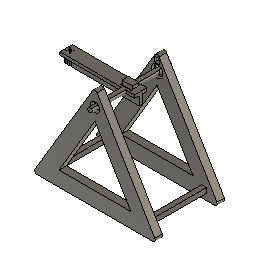
FLYArm-1D (Autodesk Fusion 360 design; units mm, degrees)
Autodesk Fusion 360 part; units mm, degrees
sketch "Szkic1" plane through (0, 0, 0) normal (0, 1, 0) x (1, 0, 0) in component "Base"
  line L0 (0, 0) -> (-250, 0)
  line L1 (-250, 0) -> (-250, -210)
  line L2 (-250, -210) -> (0, -210)
  line L3 (0, -210) -> (0, 0)
  line L4 (-250, 0) -> (-125, -210)
  line L5 (0, 0) -> (-125, -210)
  line L6 (-197.2304, -30) -> (-125, -151.3471)
  line L7 (-52.7696, -30) -> (-125, -151.3471)
  line L8 (-52.7696, -30) -> (-197.2304, -30)
  circle A0 centre (-125, -200.2245) radius 5
  circle A1 centre (-8.7949, -5) radius 5
  circle A2 centre (-241.2051, -5) radius 5
  circle A3 centre (-125, -175.7858) radius 12.025
  line L9 (-197.2304, -30) -> (-241.2051, -5)
  line L10 (-214.2178, -12.5) -> (-224.2178, -12.5)
  line L11 (-224.2178, -12.5) -> (-224.2178, -22.5)
  line L12 (-224.2178, -22.5) -> (-214.2178, -22.5)
  line L13 (-214.2178, -22.5) -> (-214.2178, -12.5)
  line L14 (-214.2178, -12.5) -> (-224.2178, -22.5) construction
  line L15 (-224.2178, -12.5) -> (-214.2178, -22.5) construction
  line L16 (-52.7696, -30) -> (-8.7949, -5)
  line L17 (-25.7822, -22.5) -> (-35.7822, -22.5)
  line L18 (-35.7822, -22.5) -> (-35.7822, -12.5)
  line L19 (-35.7822, -12.5) -> (-25.7822, -12.5)
  line L20 (-25.7822, -12.5) -> (-25.7822, -22.5)
  line L21 (-25.7822, -22.5) -> (-35.7822, -12.5) construction
  line L22 (-35.7822, -22.5) -> (-25.7822, -12.5) construction
  circle A4 centre (-125, -175.7858) radius 9.525
  line L23 (-125, -175.7858) -> (-112.975, -175.7858)
  line L24 (-125, -175.7858) -> (-137.025, -175.7858)
  line L25 (-125, -200.2245) -> (-125, -195.2245)
  line L26 (-125, -195.2245) -> (-125, -194.2245)
  line L27 (-120, -189.2245) -> (-130, -189.2245)
  line L28 (-130, -189.2245) -> (-130, -199.2245)
  line L29 (-130, -199.2245) -> (-120, -199.2245)
  line L30 (-120, -199.2245) -> (-120, -189.2245)
  line L31 (-120, -189.2245) -> (-130, -199.2245) construction
  line L32 (-130, -189.2245) -> (-120, -199.2245) construction
  point P0 (-219.2178, -17.5)
  point P1 (-30.7822, -17.5)
  point P2 (-125, -194.2245)
  point P3 (-125, -194.2245)
  dimension "d1" = 250
  dimension "d2" = 210
  dimension "d7" = 5
  dimension "d8" = 5
  dimension "d9" = 5
  dimension "d18" = 24.05
  dimension "d19" = 10
  dimension "d20" = 10
  dimension "d21" = 10
  dimension "d22" = 10
  dimension "d28" = 19.05
  dimension "d115" = 1
  dimension "d121" = 10
  dimension "d122" = 10
  constraint horizontal L0
  constraint vertical L1
  constraint horizontal L2
  constraint vertical L3
  constraint coincident L0.start L3.end
  constraint midpoint L2 L4.end
  constraint tangent L4 A0
  constraint tangent L5 A0
  constraint tangent L0 A1
  constraint tangent L5 A1
  constraint tangent L4 A2
  constraint tangent L0 A2
  constraint coincident A2.centre L9.end
  constraint horizontal L10
  constraint perpendicular L10 L11
  constraint parallel L10 L12
  constraint parallel L11 L13
  constraint coincident L14 P0
  constraint coincident L15 P0
  constraint midpoint L9 P0
  constraint coincident A1.centre L16.end
  constraint horizontal L17
  constraint perpendicular L17 L18
  constraint parallel L17 L19
  constraint parallel L18 L20
  constraint coincident L21 P1
  constraint coincident L22 P1
  constraint midpoint L16 P1
  constraint concentric A3 A4
  constraint coincident A3.centre A4.centre
  constraint coincident A3 L23.end
  constraint coincident A3 L24.end
  constraint coincident A0.centre L25.start
  constraint coincident A0 L25.end
  constraint vertical L25
  constraint parallel L25 L26
  constraint coincident P3 P2
  constraint horizontal L27
  constraint perpendicular L27 L28
  constraint parallel L27 L29
  constraint parallel L28 L30
  constraint coincident L31 P3
  constraint coincident L32 P3
  measures "d1" distance of L0.start L0.end
  measures "d2" distance of L0.start L2.end
  measures "d7" radius of A0
  measures "d8" radius of A1
  measures "d9" radius of A2
  measures "d18" diameter of A3
  measures "d19" distance of L11.end L12.end
  measures "d20" distance of L10.end L11.end
  measures "d21" distance of L18.end L19.end
  measures "d22" distance of L17.end L18.end
  measures "d28" diameter of A4
  measures "d115" distance of L25.end P3
  measures "d121" distance of L28.end L29.end
  measures "d122" distance of L27.end L28.end
extrude "Wyciągnięcie proste4" add sketch "Szkic1" against normal blind 10 contours L0 L8 A1 A2 L9 L10 L11 L13 L16 L18 L19 L20 | A1 | L4 L5 L6 L7 A0 A1 A2 L9 L11 L12 L13 L16 L17 L18 L20 L27 L28 L29 L30 | A2 | A0 L29 | L16 L17 L18 L20 | L16 L18 L19 L20 | A0 L27 L28 L29 L30 | A0 L25 L29 | A0 L25 L29 | L9 L10 L11 L13 | L9 L11 L12 L13 | A3 A4 L23 L24 | A3 A4 L23 L24 | A4 L23 L24 | A4 L23 L24 makes body 1 in component "Base"
extrude "Wyciągnięcie proste5" cut sketch "Szkic1" against normal blind 7 contours L16 L17 L18 L20 | L16 L18 L19 L20 | A0 L27 L28 L29 L30 | A0 L25 L29 | A0 L25 L29 | L9 L10 L11 L13 | L9 L11 L12 L13 | A3 A4 L23 L24 | A3 A4 L23 L24 bodies 1 in component "Base"
extrude "Wyciągnięcie proste6" cut sketch "Szkic1" against normal blind 10 contours A4 L23 L24 | A4 L23 L24 bodies 1 in component "Base"
sketch "Szkic1 (2)" plane through (0, 0, 0) normal (0, 0, 1) x (1, 0, 0) in component "Connector"
  line L0 (0, 0) -> (9.9, 0)
  line L1 (9.9, 0) -> (9.9, 124)
  line L2 (9.9, 124) -> (0, 124)
  line L3 (0, 124) -> (0, 0)
  dimension "d41" = 9.9
  dimension "d42" = 124
  constraint horizontal L0
  constraint vertical L1
  constraint horizontal L2
  constraint vertical L3
  constraint coincident L0.start L3.end
  measures "d41" distance of L0.start L0.end
  measures "d42" distance of L0.start L2.end
extrude "Wyciągnięcie proste1" add sketch "Szkic1 (2)" along normal blind 9.9 separate body makes body 2 in component "Connector"
other "Zależność geometryczna4"
other "Zależność geometryczna5"
other "Zależność geometryczna6"
other "Zależność geometryczna7"
other "Zależność geometryczna8"
other "Zależność geometryczna9"
sketch "Szkic1 (3)" plane through (0, 0, 0) normal (0, 1, 0) x (1, 0, 0) in component "Base2"
  line L0 (0, 0) -> (-250, 0)
  line L1 (-250, 0) -> (-250, -210)
  line L2 (-250, -210) -> (0, -210)
  line L3 (0, -210) -> (0, 0)
  line L4 (0, 0) -> (-125, -210)
  line L5 (-125, -210) -> (-250, 0)
  line L6 (-52.7696, -30) -> (-125, -151.3471)
  line L7 (-125, -151.3471) -> (-197.2304, -30)
  line L8 (-52.7696, -30) -> (-197.2304, -30)
  circle A0 centre (-125, -200.2245) radius 5
  circle A1 centre (-241.2051, -5) radius 5
  circle A2 centre (-8.7949, -5) radius 5
  line L9 (-241.2051, -5) -> (-197.2304, -30)
  line L10 (-8.7949, -5) -> (-52.7696, -30)
  circle A3 centre (-125, -175.7858) radius 12.025
  circle A4 centre (-125, -175.7858) radius 9.525
  line L11 (-35.7822, -12.5) -> (-25.7822, -12.5)
  line L12 (-25.7822, -12.5) -> (-25.7822, -22.5)
  line L13 (-25.7822, -22.5) -> (-35.7822, -22.5)
  line L14 (-35.7822, -22.5) -> (-35.7822, -12.5)
  line L15 (-35.7822, -12.5) -> (-25.7822, -22.5) construction
  line L16 (-25.7822, -12.5) -> (-35.7822, -22.5) construction
  line L17 (-224.2178, -22.5) -> (-214.2178, -22.5)
  line L18 (-214.2178, -22.5) -> (-214.2178, -12.5)
  line L19 (-214.2178, -12.5) -> (-224.2178, -12.5)
  line L20 (-224.2178, -12.5) -> (-224.2178, -22.5)
  line L21 (-224.2178, -22.5) -> (-214.2178, -12.5) construction
  line L22 (-214.2178, -22.5) -> (-224.2178, -12.5) construction
  line L23 (-125, -200.2245) -> (-125, -195.2245)
  line L24 (-125, -195.2245) -> (-125, -194.2245)
  line L25 (-130, -189.2245) -> (-120, -189.2245)
  line L26 (-120, -189.2245) -> (-120, -199.2245)
  line L27 (-120, -199.2245) -> (-130, -199.2245)
  line L28 (-130, -199.2245) -> (-130, -189.2245)
  line L29 (-130, -189.2245) -> (-120, -199.2245) construction
  line L30 (-120, -189.2245) -> (-130, -199.2245) construction
  point P0 (-30.7822, -17.5)
  point P1 (-219.2178, -17.5)
  point P2 (-125, -194.2245)
  dimension "d54" = 250
  dimension "d55" = 210
  dimension "d57" = 5
  dimension "d58" = 5
  dimension "d59" = 5
  dimension "d60" = 24.05
  dimension "d61" = 19.05
  dimension "d65" = 10
  dimension "d66" = 10
  dimension "d67" = 10
  dimension "d68" = 10
  dimension "d118" = 1
  dimension "d119" = 10
  dimension "d120" = 10
  constraint horizontal L0
  constraint vertical L1
  constraint horizontal L2
  constraint vertical L3
  constraint coincident L0.start L3.end
  constraint midpoint L2 L4.end
  constraint tangent L4 A0
  constraint tangent L5 A0
  constraint tangent L5 A1
  constraint tangent L0 A1
  constraint tangent L0 A2
  constraint tangent L4 A2
  constraint coincident A1.centre L9.start
  constraint coincident A2.centre L10.start
  constraint concentric A3 A4
  constraint horizontal L11
  constraint perpendicular L11 L12
  constraint parallel L11 L13
  constraint parallel L12 L14
  constraint coincident L15 P0
  constraint coincident L16 P0
  constraint midpoint L10 P0
  constraint horizontal L17
  constraint perpendicular L17 L18
  constraint parallel L17 L19
  constraint parallel L18 L20
  constraint coincident L21 P1
  constraint coincident L22 P1
  constraint midpoint L9 P1
  constraint coincident A0.centre L23.start
  constraint coincident A0 L23.end
  constraint vertical L23
  constraint parallel L23 L24
  constraint horizontal L25
  constraint perpendicular L25 L26
  constraint parallel L25 L27
  constraint parallel L26 L28
  constraint coincident L29 P2
  constraint coincident L30 P2
  constraint coincident P2 L24.end
  measures "d54" distance of L0.start L0.end
  measures "d55" distance of L0.start L2.end
  measures "d57" radius of A0
  measures "d58" radius of A1
  measures "d59" radius of A2
  measures "d60" diameter of A3
  measures "d61" diameter of A4
  measures "d65" distance of L12.end L13.end
  measures "d66" distance of L11.end L12.end
  measures "d67" distance of L18.end L19.end
  measures "d68" distance of L17.end L18.end
  measures "d118" distance of L23.end P2
  measures "d119" distance of L26.end L27.end
  measures "d120" distance of L25.end L26.end
  measures "d221" distance of L0.start
extrude "Wyciągnięcie proste1'" add sketch "Szkic1 (3)" along normal blind 10 separate body contours L0 L8 A1 A2 L9 L10 L11 L12 L14 L18 L19 L20 | A2 | L4 L5 L6 L7 A0 A1 A2 L9 L10 L12 L13 L14 L17 L18 L20 L25 L26 L27 L28 | A1 | A0 L27 | L10 L12 L13 L14 | L10 L11 L12 L14 | A0 L25 L26 L27 L28 | A0 L23 L27 | A0 L23 L27 | L9 L18 L19 L20 | L9 L17 L18 L20 | A3 | A4 makes body 3 in component "Base2"
extrude "Wyciągnięcie proste2" cut sketch "Szkic1 (3)" along normal blind 7 contours L10 L12 L13 L14 | L10 L11 L12 L14 | A0 L25 L26 L27 L28 | A0 L23 L27 | A0 L23 L27 | L9 L18 L19 L20 | L9 L17 L18 L20 | A3 bodies 3 in component "Base2"
extrude "Wyciągnięcie proste3" cut sketch "Szkic1 (3)" along normal blind 10 contours A4 bodies 3 in component "Base2"
other "Zależność geometryczna10"
other "Zależność geometryczna11"
other "Zależność geometryczna12"
ref_plane "Płaszczyzna konstrukcyjna1" through (-125, 0, 175.7858) normal (1, 0, 0) x (0, 1, 0) in component "Bar"
sketch "Szkic1 (4)" plane through (-125, 0, 175.7858) normal (1, 0, 0) x (0, 1, 0) in component "Bar"
  line L0 (0, 0) -> (95, 0)
  line L1 (47.5, 0) -> (60, 0)
  line L2 (47.5, 0) -> (35, 0)
  line L3 (60, 0) -> (60, -6)
  line L4 (35, 0) -> (35, -6)
  line L5 (47.5, 0) -> (47.5, -24)
  line L6 (47.5, -24) -> (50.5, -24)
  line L7 (47.5, -24) -> (44.5, -24)
  line L8 (50.5, -24) -> (50.5, -6)
  line L9 (44.5, -24) -> (44.5, -6)
  line L10 (35, -6) -> (44.5, -6)
  line L11 (60, -6) -> (50.5, -6)
  line L12 (95, 0) -> (95, -175.786)
  line L13 (0, 0) -> (0, -175.786)
  line L14 (0, -175.786) -> (95, -175.786)
  line L15 (47.5, -175.786) -> (47.5, -165.786)
  line L16 (47.5, -165.786) -> (47.5, -120.786)
  line L17 (47.5, -120.786) -> (47.5, 0)
  dimension "d82" = 12.5
  dimension "d83" = 12.5
  dimension "d85" = 6
  dimension "d86" = 6
  dimension "d91" = 24
  dimension "d92" = 3
  dimension "d93" = 3
  dimension "d94" = 18
  dimension "d95" = 18
  dimension "d99" = 175.786
  dimension "d100" = 175.786
  dimension "d102" = 10
  dimension "d103" = 45
  dimension "d104" = 120.786
  constraint coincident L0.start L13.start
  constraint horizontal L0
  constraint midpoint L0 L1.start
  constraint parallel L0 L1
  constraint parallel L0 L2
  constraint perpendicular L0 L3
  constraint perpendicular L2 L4
  constraint perpendicular L1 L5
  constraint perpendicular L5 L6
  constraint perpendicular L5 L7
  constraint perpendicular L6 L8
  constraint perpendicular L7 L9
  constraint perpendicular L0 L12
  constraint perpendicular L0 L13
  constraint midpoint L14 L15.start
  constraint perpendicular L14 L15
  constraint parallel L15 L16
  constraint perpendicular L2 L17
  measures "d82" distance of L1.start L1.end
  measures "d83" distance of L1.start L2.end
  measures "d85" distance of L1.end L3.end
  measures "d86" distance of L2.end L4.end
  measures "d91" distance of L1.start L5.end
  measures "d92" distance of L5.end L6.end
  measures "d93" distance of L5.end L7.end
  measures "d94" distance of L6.end L8.end
  measures "d95" distance of L7.end L9.end
  measures "d99" distance of L0.end L12.end
  measures "d100" distance of L0.start L13.end
  measures "d102" distance of L15.start L15.end
  measures "d103" distance of L15.end L16.end
  measures "d104" distance of L16.end L1.start
extrude "Wyciągnięcie proste1''" add sketch "Szkic1 (4)" against normal blind 128 separate body contours L0 L2 L4 L5 L7 L9 L10 L17 | L0 L1 L3 L5 L6 L8 L11 L17 makes body 4 in component "Bar"
sketch "Szkic2" plane through (0, 0, 175.7858) normal (0, 0, 1) x (-1, 0, 0) in component "Bar"
  line L0 (125, -60) -> (253, -60)
  line L1 (253, -60) -> (253, -35)
  line L2 (253, -35) -> (125, -35)
  line L3 (125, -47.5) -> (245, -47.5)
  line L4 (249.2425, -51.7425) -> (240.7575, -51.7425)
  line L5 (240.7575, -51.7425) -> (240.7575, -43.2575)
  line L6 (240.7575, -43.2575) -> (249.2425, -43.2575)
  line L7 (249.2425, -43.2575) -> (249.2425, -51.7425)
  line L8 (249.2425, -51.7425) -> (240.7575, -43.2575) construction
  line L9 (240.7575, -51.7425) -> (249.2425, -43.2575) construction
  circle A0 centre (240.7575, -43.2575) radius 1
  circle A1 centre (249.2425, -43.2575) radius 1
  circle A2 centre (240.7575, -51.7425) radius 1
  circle A3 centre (249.2425, -51.7425) radius 1
  circle A4 centre (245, -47.5) radius 2.5
  point P0 (245, -47.5)
  dimension "d152" = 120
  dimension "d153" = 8.485
  dimension "d154" = 8.485
  dimension "d155" = 2
  dimension "d156" = 2
  dimension "d157" = 2
  dimension "d158" = 2
  dimension "d191" = 5
  constraint horizontal L4
  constraint perpendicular L4 L5
  constraint parallel L4 L6
  constraint parallel L5 L7
  constraint coincident L8 P0
  constraint coincident L9 P0
  constraint coincident P0 L3.end
  constraint coincident L5.end L6.start
  constraint coincident L6.end L7.start
  constraint coincident L4.end L5.start
  constraint coincident L4.start L7.end
  measures "d152" distance of L3.start P0
  measures "d153" distance of L5.end L6.end
  measures "d154" distance of L4.end L5.end
  measures "d155" diameter of A0
  measures "d156" diameter of A1
  measures "d157" diameter of A2
  measures "d158" diameter of A3
  measures "d191" diameter of A4
other "Zależność geometryczna16"
other "Zależność geometryczna17"
other "Zależność geometryczna18"
extrude "Wyciągnięcie proste3'" add 1 faces at (-125, 47.5, 163.7858) along direction (1, 0, 0) blind 12.025 on bodies 4 bodies 4 in component "Bar"
ref_plane "Płaszczyzna konstrukcyjna2" through (-182.9875, 47.5, 172.7858) normal (0, 1, 0) x (0, 0, -1) in component "Bar"
sketch "Szkic5" plane through (0, 47.5, 0) normal (0, 1, 0) x (1, 0, 0) in component "Bar"
extrude "Wyciągnięcie proste8" cut sketch "Szkic2" against normal blind 36 contours L4 L5 A2 | L4 L5 A2 | L4 L7 A3 | L4 L7 A3 | L6 L7 A1 | L6 L7 A1 | L5 L6 A0 | L5 L6 A0 bodies 4 in component "Bar"
sketch "Szkic6" plane through (0, 50.5, 0) normal (0, 1, 0) x (-1, 0, 0) in component "Bar"
  line L0 (112.975, 151.7858) -> (253, 151.7858)
  line L1 (253, 151.7858) -> (253, 169.7858)
  line L2 (253, 169.7858) -> (112.975, 169.7858)
  line L3 (112.975, 169.7858) -> (112.975, 151.7858)
  line L4 (112.975, 169.7858) -> (125, 169.7858)
  line L5 (125, 169.7858) -> (125, 176.7858)
  line L6 (125, 169.7858) -> (125, 159.7858)
  circle A0 centre (125, 172.3108) radius 4.475
  line L7 (125, 176.7858) -> (125, 175.7858)
  line L8 (125, 175.7858) -> (122.1804, 175.7858)
  line L9 (125, 175.7858) -> (127.8196, 175.7858)
  line L10 (125, 176.7858) -> (125, 172.3108)
  circle A1 centre (125, 172.3108) radius 5.475
  line L11 (122.1804, 175.7858) -> (120.7692, 175.7858)
  line L12 (127.8196, 175.7858) -> (129.2308, 175.7858)
  dimension "d161" = 12.025
  dimension "d162" = 7
  dimension "d163" = 10
  dimension "d164" = 8.95
  dimension "d169" = 1
  dimension "d198" = 4.475
  dimension "d199" = 10.95
  constraint coincident L2.end L3.start
  constraint coincident L2 L4.end
  constraint perpendicular L2 L5
  constraint perpendicular L4 L6
  constraint coincident L5.end A0
  constraint parallel L5 L7
  constraint coincident A0 L8.end
  constraint perpendicular L7 L8
  constraint coincident A0 L9.end
  constraint perpendicular L7 L9
  constraint parallel L5 L10
  constraint concentric A0 A1
  constraint coincident A1 L11.end
  constraint parallel L8 L11
  constraint coincident A1 L12.end
  constraint parallel L9 L12
  measures "d161" distance of L2.end L4.end
  measures "d162" distance of L4.end L5.end
  measures "d163" distance of L4.end L6.end
  measures "d164" diameter of A0
  measures "d169" distance of L5.end L7.end
  measures "d198" distance of L5.end A0.centre
  measures "d199" diameter of A1
sketch "Szkic7" plane through (0, 44.5, 0) normal (0, -1, 0) x (1, 0, 0) in component "Bar"
  line L0 (-112.975, 169.7858) -> (-253, 169.7858)
  line L1 (-253, 169.7858) -> (-253, 151.7858)
  line L2 (-253, 151.7858) -> (-112.975, 151.7858)
  line L3 (-112.975, 151.7858) -> (-112.975, 169.7858)
  line L4 (-112.975, 169.7858) -> (-125, 169.7858)
  line L5 (-125, 169.7858) -> (-125, 176.7858)
  line L6 (-125, 169.7858) -> (-125, 159.7858)
  circle A0 centre (-125, 172.3108) radius 4.475
  line L7 (-125, 176.7858) -> (-125, 175.7858)
  line L8 (-125, 175.7858) -> (-122.1804, 175.7858)
  line L9 (-125, 175.7858) -> (-127.8196, 175.7858)
  line L10 (-125, 176.7858) -> (-125, 172.3108)
  circle A1 centre (-125, 172.3108) radius 5.475
  line L11 (-127.8196, 175.7858) -> (-129.2308, 175.7858)
  line L12 (-122.1804, 175.7858) -> (-120.7692, 175.7858)
  dimension "d165" = 12.025
  dimension "d166" = 7
  dimension "d167" = 10
  dimension "d168" = 8.95
  dimension "d170" = 1
  dimension "d202" = 4.475
  dimension "d203" = 10.95
  constraint coincident L0.start L3.end
  constraint perpendicular L3 L4
  constraint perpendicular L4 L5
  constraint perpendicular L4 L6
  constraint coincident L5.end A0
  constraint parallel L5 L7
  constraint coincident A0 L8.end
  constraint perpendicular L5 L8
  constraint coincident A0 L9.end
  constraint perpendicular L7 L9
  constraint perpendicular L8 L10
  constraint coincident A0.centre L10.end
  constraint coincident A1 L11.end
  constraint parallel L9 L11
  constraint coincident A1 L12.end
  constraint parallel L8 L12
  measures "d165" distance of L0.start L4.end
  measures "d166" distance of L4.end L5.end
  measures "d167" distance of L4.end L6.end
  measures "d168" diameter of A0
  measures "d170" distance of L5.end L7.end
  measures "d202" distance of L5.end A0.centre
  measures "d203" diameter of A1
extrude "Wyciągnięcie proste9" add sketch "Szkic7" along normal blind 77 contours L0 L4 L6 A0 | L0 L4 L5 A0 L8 L10 | L0 L6 A0 | L0 L5 A0 L9 L10 bodies 4 in component "Bar"
extrude "Wyciągnięcie proste10" add sketch "Szkic6" along normal blind 77 contours L2 L4 L5 A0 L8 L10 | L2 L4 L6 A0 | L2 L6 A0 | L2 L5 A0 L9 L10 bodies 4 in component "Bar"
sketch "Szkic11" plane through (0, 127.5, 0) normal (0, 1, 0) x (-1, 0, 0) in component "Bar"
  arc A0 (122.1804, 175.7858) -> (127.8196, 175.7858) centre (125, 172.3108) ccw
  line L0 (127.8196, 175.7858) -> (122.1804, 175.7858)
  circle A1 centre (125, 172.3108) radius 12.025
  line L1 (125, 172.3108) -> (125, 160.2858)
  line L2 (125, 172.3108) -> (125, 151)
  line L3 (125, 175.7858) -> (125, 169.7858)
  line L4 (125, 169.7858) -> (110.6889, 169.7858)
  line L5 (110.6889, 169.7858) -> (110.6889, 143)
  line L6 (125, 151) -> (105, 151)
  dimension "d181" = 24.05
  dimension "d182" = 6
  constraint concentric A0 A1
  constraint coincident A0.centre A1.centre
  constraint coincident A1 L1.end
  constraint vertical L1
  constraint parallel L1 L2
  constraint midpoint L0 L3.start
  constraint perpendicular L0 L3
  constraint perpendicular L1 L4
  constraint perpendicular L4 L5
  constraint perpendicular L2 L6
  measures "d181" diameter of A1
  measures "d182" distance of L3.start L3.end
extrude "Wyciągnięcie proste7" add 1 faces at (-149.0768, -10, 10) along direction (0, -1, 0) blind 5 on bodies 1 bodies 1 in component "Base"
extrude "Wyciągnięcie proste4'" add 1 faces at (-149.0768, 10, 10) along direction (0, 1, 0) blind 5 on bodies 3 bodies 3 in component "Base2"
other "Zależność geometryczna22"
extrude "Wyciągnięcie proste13" cut sketch "Szkic2" against normal blind 2 contours A4 bodies 4 in component "Bar"
sketch "Szkic12" plane through (0, 0, 175.7858) normal (0, 0, 1) x (-1, 0, 0) in component "Bar"
  circle A0 centre (245, -47.5) radius 2.5
  circle A1 centre (249.2425, -43.2575) radius 1
  circle A2 centre (240.7575, -43.2575) radius 1
  circle A3 centre (249.2425, -51.7425) radius 1
  circle A4 centre (240.7575, -51.7425) radius 1
  line L0 (127.8196, -60) -> (253, -60)
  line L1 (253, -60) -> (253, -35)
  line L2 (253, -35) -> (127.8196, -35)
  line L3 (127.8196, -35) -> (127.8196, 32.5)
  line L4 (127.8196, 32.5) -> (122.1804, 32.5)
  line L5 (122.1804, 32.5) -> (122.1804, -35)
  line L6 (122.1804, -35) -> (112.975, -35)
  line L7 (112.975, -35) -> (112.975, -60)
  line L8 (112.975, -60) -> (122.1804, -60)
  line L9 (122.1804, -60) -> (122.1804, -127.5)
  line L10 (122.1804, -127.5) -> (127.8196, -127.5)
  line L11 (127.8196, -127.5) -> (127.8196, -60)
  line L12 (122.1804, -35) -> (127.8196, -35)
  line L13 (122.1804, -35) -> (122.1804, -60)
  line L14 (125, -35) -> (125, -52.3294)
  line L15 (122.1804, -47.5) -> (129.8919, -47.5)
  line L16 (135.5, -39.5) -> (114.5, -39.5)
  line L17 (114.5, -39.5) -> (114.5, -55.5)
  line L18 (114.5, -55.5) -> (135.5, -55.5)
  line L19 (135.5, -55.5) -> (135.5, -39.5)
  line L20 (135.5, -39.5) -> (114.5, -55.5) construction
  line L21 (114.5, -39.5) -> (135.5, -55.5) construction
  point P0 (125, -47.5)
  dimension "d194" = 21
  dimension "d195" = 16
  constraint coincident L5.end L6.start
  constraint coincident L2.end L3.start
  constraint coincident L8.end L9.start
  constraint midpoint L12 L14.start
  constraint perpendicular L12 L14
  constraint midpoint L13 L15.start
  constraint perpendicular L13 L15
  constraint horizontal L16
  constraint perpendicular L16 L17
  constraint parallel L16 L18
  constraint parallel L17 L19
  constraint coincident L20 P0
  constraint coincident L21 P0
  constraint coincident L14 P0
  constraint coincident L15 P0
  measures "d194" distance of L17.end L18.end
  measures "d195" distance of L16.end L17.end
extrude "Wyciągnięcie proste14" add 1 faces at (-112.975, 46.5, 173.7858) along direction (1, 0, 0) blind 10 on bodies 4 bodies 4 in component "Bar"
extrude "Wyciągnięcie proste15" add sketch "Szkic6" along normal blind 52 contours L2 L4 A0 A1 L11 | L2 L4 L6 A0 A1 | L2 L6 A0 A1 | L2 A0 A1 L12 bodies 4 in component "Bar"
extrude "Wyciągnięcie proste16" add sketch "Szkic7" along normal blind 52 contours L0 L4 L6 A0 A1 | L0 L4 A0 A1 L12 | L0 L6 A0 A1 | L0 A0 A1 L11 bodies 4 in component "Bar"
other "Zależność geometryczna23"
sketch "Szkic13" plane through (0, 0, 169.7858) normal (0, 0, -1) x (1, 0, 0) in component "Bar"
  line L0 (-129.858, -60) -> (-129.858, -50.5)
  line L1 (-129.858, -50.5) -> (-253, -50.5)
  line L2 (-253, -50.5) -> (-253, -60)
  line L3 (-253, -60) -> (-129.858, -60)
  circle A0 centre (-249.2425, -51.7425) radius 1
  circle A1 centre (-240.7575, -51.7425) radius 1
  circle A2 centre (-240.7575, -51.7425) radius 2.5
  circle A3 centre (-249.2425, -51.7425) radius 2.5
  line L4 (-249.2425, -51.7425) -> (-240.7572, -43.2572)
  line L5 (-249.2425, -51.7425) -> (-237.2425, -51.7425) construction
  circle A4 centre (-240.7572, -43.2572) radius 2.5
  line L6 (-240.7575, -51.7425) -> (-249.2428, -43.2572)
  line L7 (-240.7575, -51.7425) -> (-252.7575, -51.7425) construction
  circle A5 centre (-249.2428, -43.2572) radius 2.5
  dimension "d207" = 5
  dimension "d208" = 5
  dimension "d209" = 45
  dimension "d210" = 12
  dimension "d211" = 5
  dimension "d212" = 45
  dimension "d213" = 12
  dimension "d214" = 5
  constraint concentric A1 A2
  constraint concentric A0 A3
  constraint horizontal L5
  constraint coincident A0.centre A3.centre
  constraint coincident L4.end A4.centre
  constraint horizontal L7
  constraint coincident A1.centre A2.centre
  constraint coincident L6.end A5.centre
  measures "d207" diameter of A2
  measures "d208" diameter of A3
  measures "d209" angle of L4 L5
  measures "d210" distance of A0.centre L4.end
  measures "d211" diameter of A4
  measures "d212" angle of L6 L7
  measures "d213" distance of A1.centre L6.end
  measures "d214" diameter of A5
extrude "Wyciągnięcie proste17" cut sketch "Szkic13" along normal blind 30 contours L1 A2 | L1 A2 L6 | L1 A2 L6 | L1 A3 L4 | L1 A3 | L1 A3 L4 | A4 | A5 bodies 4 in component "Bar"
extrude "Wyciągnięcie proste18" cut sketch "Szkic13" against normal blind 1.7 contours L1 A2 | L1 A2 L6 | L1 A2 L6 | L1 A3 L4 | L1 A3 | L1 A3 L4 | A4 | A5 bodies 4 in component "Bar"
extrude "Wyciągnięcie proste19" cut sketch "Szkic12" against normal blind 2 contours L13 L16 L17 L18 | L13 L14 L15 L16 L18 L19 | L13 L14 L15 L16 bodies 4 in component "Bar"
sketch "Szkic14" plane through (0, 0, 173.7858) normal (0, 0, 1) x (-1, 0, 0) in component "Bar"
  line L0 (135.5, -55.5) -> (135.5, -39.5)
  line L1 (135.5, -39.5) -> (114.5, -39.5)
  line L2 (114.5, -39.5) -> (114.5, -55.5)
  line L3 (114.5, -55.5) -> (135.5, -55.5)
  line L4 (114.5, -39.5) -> (135.5, -39.5)
  line L5 (135.5, -39.5) -> (135.5, -55.5)
  line L6 (135.5, -55.5) -> (114.5, -55.5)
  line L7 (114.5, -55.5) -> (114.5, -39.5)
  line L8 (125, -39.5) -> (125, -55.5)
  line L9 (125, -55.5) -> (125, -49)
  line L10 (135.35, -55.5) -> (114.65, -55.5)
  line L11 (114.65, -55.5) -> (114.65, -42.5)
  line L12 (114.65, -42.5) -> (135.35, -42.5)
  line L13 (135.35, -42.5) -> (135.35, -55.5)
  line L14 (135.35, -55.5) -> (114.65, -42.5) construction
  line L15 (114.65, -55.5) -> (135.35, -42.5) construction
  point P0 (125, -49)
  dimension "d221" = 6.5
  dimension "d222" = 20.7
  dimension "d223" = 13
  constraint horizontal L4
  constraint vertical L5
  constraint horizontal L6
  constraint vertical L7
  constraint coincident L0.start L3.end
  constraint coincident L1.end L2.start
  constraint midpoint L4 L8.start
  constraint midpoint L6 L8.end
  constraint perpendicular L6 L9
  constraint horizontal L10
  constraint perpendicular L10 L11
  constraint parallel L10 L12
  constraint parallel L11 L13
  constraint coincident L14 P0
  constraint coincident L15 P0
  constraint coincident P0 L9.end
  measures "d221" distance of L8.end P0
  measures "d222" distance of L11.end L12.end
  measures "d223" distance of L10.end L11.end
extrude "Wyciągnięcie proste20" add sketch "Szkic14" along normal blind 8 separate body contours L3 L6 L8 L9 L10 L12 L13 | L3 L6 L8 L9 L10 L11 L12 makes body 5 in component "Bar"
component "Base" placed x (1, 0, 0) y (0, 1, 0) z (0, 0, 1) at (0, 0, 0)
component "Connector" placed x (1, 0, 0) y (0, 1, 0) z (0, 0, 1) at (-35.6822, -7, 12.6)
component "Connector" placed x (1, 0, 0) y (0, 1, 0) z (0, 0, 1) at (-224.1178, -7, 12.6)
component "Connector" placed x (1, 0, 0) y (0, 1, 0) z (0, 0, 1) at (-130, -7, 189.2245)
component "Base2" placed x (1, 0, 0) y (0, 1, 0) z (0, 0, 1) at (0, 110, 0.1)
component "Bar" placed x (0.999998, 0, -0.002052) y (0, 1, 0) z (0.002052, 0, 0.999998) at (-0.3538, 7.5, 3.2189)
equation "thick = 30 mm"
equation "socket = 24.05 mm"
equation "connectionSocket = 10 mm"
equation "d6 = -thick"
equation "frameHeight = 10 mm"
equation "d18 = socket"
equation "d19 = connectionSocket"
equation "d20 = connectionSocket"
equation "d21 = connectionSocket"
equation "d22 = connectionSocket"
equation "socketIns = socket - 5 mm"
equation "d28 = socketIns"
equation "d29 = -frameHeight"
equation "d33 = -frameHeight"
equation "frameGap = 110 mm"
equation "connectorOffset = 0.1 mm"
equation "d41 = connectionSocket - connectorOffset"
equation "d42 = frameGap + 14 mm"
equation "d43 = connectionSocket - connectorOffset"
equation "d56 = -thick"
equation "d60 = socket"
equation "d61 = socketIns"
equation "d65 = connectionSocket"
equation "d66 = connectionSocket"
equation "d67 = connectionSocket"
equation "d68 = connectionSocket"
equation "d69 = frameHeight"
equation "d73 = frameHeight"
equation "barWidth = 25 mm"
equation "barHeight = 6 mm"
equation "d82 = barWidth / 2"
equation "d83 = barWidth / 2"
equation "d85 = barHeight"
equation "d86 = barHeight"
equation "d91 = barHeight * 4"
equation "d92 = barHeight / 2"
equation "d93 = barHeight / 2"
equation "d94 = barHeight * 3"
equation "d95 = barHeight * 3"
equation "barLength = 128 mm"
equation "d97 = -barLength"
equation "d119 = connectionSocket"
equation "d120 = connectionSocket"
equation "d121 = connectionSocket"
equation "d122 = connectionSocket"
equation "d129 = socket / 2"
equation "stick = 8.95 mm"
equation "d151 = -barWidth / 2"
equation "d161 = socket / 2"
equation "d162 = barHeight + 1 mm"
equation "d164 = stick"
equation "d165 = socket / 2"
equation "d166 = barHeight + 1 mm"
equation "d168 = stick"
equation "d171 = ( 140 / 2 ) * 1 mm - 3 mm + 10 mm"
equation "d173 = ( 140 / 2 ) * 1 mm - 3 mm + 10 mm"
equation "d181 = socket"
equation "d198 = stick / 2"
equation "d199 = stick + 2 mm"
equation "d200 = 42.5 mm + 9.5 mm"
equation "d202 = stick / 2"
equation "d203 = stick + 2 mm"
equation "d204 = 42.5 mm + 9.5 mm"
equation "d217 = -6 mm + 4.3 mm"
equation "d221 = ( 13 / 2 ) * 1 mm"
equation "d222 = 21 mm - 0.3 mm"
named bodies: "BaseRight", "BaseLeft", "Bar", "MpuHolder"
